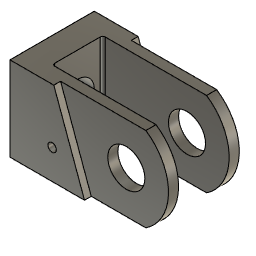
Ejercicio01_jaalobuela (Autodesk Fusion 360 design; units mm, degrees)
Autodesk Fusion 360 part; units mm, degrees
note: some values were not read from the file. Set by a fixed rule: which sketch regions a step uses.
sketch "Sketch1" plane through (0, 0, 0) normal (0, 1, 0) x (1, 0, 0)
  line L0 (50, -50) -> (50, 0)
  line L1 (50, 0) -> (115, 0)
  line L2 (50, -50) -> (115, -50)
  circle A0 centre (115, -25) radius 11
  line L3 (115, -50) -> (126.5831, -50)
  line L4 (150, -50) -> (150, -51.6194)
  line L5 (115, 0) -> (126.5831, 0)
  line L6 (50, -50) -> (50, -57.444) construction
  line L7 (50, -57.444) -> (76, -57.444) construction
  line L8 (76, -57.444) -> (76, 0) construction
  line L9 (76, -50) -> (94.1985, 0)
  line L10 (50, 0) -> (126.5831, 0) construction
  line L11 (140, 0) -> (140, -25) construction
  arc A1 (126.5831, -50) -> (126.5831, 0) centre (110, -25) ccw
  dimension "d1" = 50
  dimension "d2" = 65
  dimension "d3" = 65
  dimension "d4" = 22
  dimension "d6" = 1.6194
  dimension "d7" = 26
  dimension "d8" = 110
  dimension "d37" = 90
  dimension "d38" = 60
  constraint vertical L0
  constraint perpendicular L0 L1
  constraint perpendicular L0 L2
  constraint perpendicular L2 L4
  constraint perpendicular L2 L6
  constraint perpendicular L6 L7
  constraint coincident L1 L8.end
  constraint perpendicular L1 L8
  constraint coincident L2 L9.start
  constraint coincident L8 L9.start
  constraint coincident L1 L9.end
  constraint perpendicular L0 L10
  constraint perpendicular L10 L11
  measures "d1" distance of L0.start L0.end
  measures "d2" distance of L0.end L1.end
  measures "d3" distance of L0.start L2.end
  measures "d4" diameter of A0
  measures "d6" distance of L4.start L4.end
  measures "d7" distance of L6.end L7.end
  measures "d8" angle of L1 L9
  measures "d37" distance of L0.end L11.start
  measures "d38" diameter of A1
extrude "Extrude1" add sketch "Sketch1" against normal blind 4 contours L0 L1 L2 L9 makes body 1
move_body "Move1" bodies 1 to x (1, 0, 0) y (0, 1, 0) z (0, 0, 1) at (0, -75, 0)
extrude "Extrude2" add sketch "Sketch1" along normal blind 6 separate body makes body 2
copy_body "CopyPasteBodies1" bodies 2 1 makes body 3 makes body 4
move_body "Move2" bodies 3 4 to x (1, 0, 0) y (0, 1, 0) z (0, 0, 1) at (0, 200, 0)
move_body "Move3" bodies 1 to x (1, 0, 0) y (0, 1, 0) z (0, 0, 1) at (0, 75, 0)
box "BoxPrimitive1" add length 50 width 50 height 15 placed x (0, 0, -1) y (0, 1, 0) z (1, 0, 0) at (0, -15, 65) separate body makes body 5
move_body "Move4" bodies 5 to x (1, 0, 0) y (0, 1, 0) z (0, 0, 1) at (50, 11, -15)
move_body "Move5" bodies 4 to x (1, 0, 0) y (0, 1, 0) z (0, 0, 1) at (0, 85, 0)
move_body "Move6" bodies 3 4 to x (1, 0, 0) y (0, 1, 0) z (0, 0, 1) at (0, -164, 0)
copy_body "CopyPasteBodies2" bodies 1 2 4 3 5 makes body 6 makes body 7 makes body 8 makes body 9 makes body 10
move_body "Move7" bodies 6 7 8 9 10 to x (1, 0, 0) y (0, 1, 0) z (0, 0, 1) at (-230, 0, 0)
combine "Combine1" operation add target body 2 tool bodies 3 4 5 1
fillet "Fillet1" radius 1.5 2 edges at (65, 6, 25) (65, 36, 25) on bodies 2
hole "Hole1" at (75, -4, 17.5) direction (0, 1, 0) diameter 5 depth 90 tip angle 118 bodies 2
hole "Hole2" at (50, 21, 25) direction (1, 0, 0) diameter 20 depth 90 tip angle 118 counterbore diameter 35 counterbore depth 2 bodies 2
hidden bodies 6 7 8 9 10
